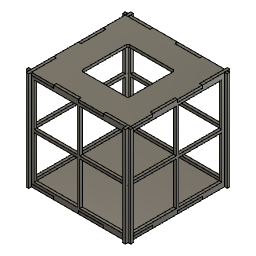
Big Switch Lamp (Autodesk Fusion 360 design; units mm, degrees)
Autodesk Fusion 360 part; units mm, degrees
note: some values were not read from the file. Chosen so that the rebuilt part matches the saved one: which bodies a step acts on.
sketch "Sketch1" plane through (0, 0, 0) normal (1, 0, 0) x (0, 0, -1) in component "Sides"
  line L0 (0, 0) -> (111.6, 0) construction
  line L1 (111.6, 0) -> (111.6, 111.6) construction
  line L2 (111.6, 111.6) -> (0, 111.6) construction
  line L3 (0, 111.6) -> (0, 0) construction
  line L4 (3.175, 108.425) -> (54.2125, 108.425)
  line L5 (54.2125, 108.425) -> (54.2125, 57.3875)
  line L6 (54.2125, 57.3875) -> (3.175, 57.3875)
  line L7 (3.175, 57.3875) -> (3.175, 108.425)
  line L8 (57.3875, 108.425) -> (108.425, 108.425)
  line L9 (108.425, 108.425) -> (108.425, 57.3875)
  line L10 (108.425, 57.3875) -> (57.3875, 57.3875)
  line L11 (57.3875, 57.3875) -> (57.3875, 108.425)
  line L12 (3.175, 54.2125) -> (54.2125, 54.2125)
  line L13 (54.2125, 54.2125) -> (54.2125, 3.175)
  line L14 (54.2125, 3.175) -> (3.175, 3.175)
  line L15 (3.175, 3.175) -> (3.175, 54.2125)
  line L16 (57.3875, 54.2125) -> (108.425, 54.2125)
  line L17 (108.425, 54.2125) -> (108.425, 3.175)
  line L18 (108.425, 3.175) -> (57.3875, 3.175)
  line L19 (57.3875, 3.175) -> (57.3875, 54.2125)
  line L20 (0, 93) -> (3.175, 93) construction
  line L21 (15, 108.425) -> (15, 111.6) construction
  line L22 (15, 57.3875) -> (15, 54.2125) construction
  line L23 (15, 3.175) -> (15, 0) construction
  line L24 (54.2125, 93) -> (57.3875, 93) construction
  line L25 (108.425, 92.9494) -> (111.6, 92.9494) construction
  line L26 (-6.35, 114.775) -> (117.95, 114.775)
  line L27 (117.95, 114.775) -> (117.95, -3.175)
  line L28 (117.95, -3.175) -> (-6.35, -3.175)
  line L29 (-6.35, -3.175) -> (-6.35, 114.775)
  line L30 (108.425, 105.4235) -> (117.95, 105.4235) construction
  line L31 (8.936, 114.775) -> (8.936, 108.425) construction
  dimension "d23" = 111.6
  dimension "d24" = 111.6
  dimension "d25" = 3.175
  dimension "d26" = 3.175
  dimension "d27" = 3.175
  dimension "d28" = 3.175
  dimension "d29" = 3.175
  dimension "d30" = 3.175
  dimension "d31" = 124.3
  dimension "d32" = 9.525
  dimension "d33" = 117.95
  dimension "d34" = 6.35
  constraint horizontal L0
  constraint vertical L1
  constraint horizontal L2
  constraint vertical L3
  constraint coincident L0.start L3.end
  constraint horizontal L4
  constraint vertical L5
  constraint horizontal L6
  constraint vertical L7
  constraint horizontal L8
  constraint vertical L9
  constraint horizontal L10
  constraint vertical L11
  constraint horizontal L12
  constraint vertical L13
  constraint horizontal L14
  constraint vertical L15
  constraint horizontal L16
  constraint vertical L17
  constraint horizontal L18
  constraint vertical L19
  constraint equal L4 L8
  constraint equal L10 L16
  constraint equal L14 L18
  constraint equal L7 L11
  constraint equal L9 L17
  constraint equal L13 L19
  constraint collinear L7 L15
  constraint collinear L11 L19
  constraint collinear L4 L8
  constraint collinear L12 L16
  constraint coincident L3 L20.start
  constraint coincident L7 L20.end
  constraint perpendicular L7 L20
  constraint coincident L4 L21.start
  constraint coincident L2 L21.end
  constraint perpendicular L2 L21
  constraint coincident L6 L22.start
  constraint coincident L12 L22.end
  constraint perpendicular L12 L22
  constraint coincident L14 L23.start
  constraint coincident L0 L23.end
  constraint perpendicular L0 L23
  constraint coincident L5 L24.start
  constraint coincident L11 L24.end
  constraint perpendicular L11 L24
  constraint coincident L9 L25.start
  constraint coincident L1 L25.end
  constraint perpendicular L1 L25
  constraint horizontal L26
  constraint vertical L27
  constraint horizontal L28
  constraint vertical L29
  constraint coincident L9 L30.start
  constraint coincident L27 L30.end
  constraint perpendicular L27 L30
  constraint coincident L26 L31.start
  constraint coincident L4 L31.end
  constraint perpendicular L4 L31
  measures "d23" distance of L0.start L2.end
  measures "d24" distance of L0.start L0.end
  measures "d25" distance of L20.start L20.end
  measures "d26" distance of L24.start L24.end
  measures "d27" distance of L25.start L25.end
  measures "d28" distance of L21.start L21.end
  measures "d29" distance of L22.start L22.end
  measures "d30" distance of L23.start L23.end
  measures "d31" distance of L27.end L28.end
  measures "d32" distance of L30.start L30.end
  measures "d33" distance of L26.start L28.end
  measures "d34" distance of L31.start L31.end
extrude "Extrude1" add sketch "Sketch1" along normal blind 3.175 makes body 1 in component "Sides"
pattern_circular "C-Pattern1" count 4 over 360 about axis through (0, -3.175, 6.35) along (0, 1, 0) of bodies 1 makes body 2 at (-121.125, 56.3292, 6.35) makes body 3 at (0, 56.3292, 127.475) makes body 4 at (121.125, 56.3292, 6.35) in component "Sides"
move_body "Move1" bodies 4 to x (1, 0, 0) y (0, 1, 0) z (0, 0, 1) at (-117.95, 0, -58.975) in component "Sides"
move_body "Move2" bodies 4 to x (1, 0, 0) y (0, 1, 0) z (0, 0, 1) at (0, 0, -62.15) in component "Sides"
move_body "Move3" bodies 2 to x (1, 0, 0) y (0, 1, 0) z (0, 0, 1) at (6.35, 0, -3.175) in component "Sides"
move_body "Move4" bodies 3 to x (1, 0, 0) y (0, 1, 0) z (0, 0, 1) at (-111.6, 0, -124.3) in component "Sides"
sketch "Sketch5" plane through (0, 0, 0) normal (0, 1, 0) x (1, 0, 0) in component "Bottom"
  line L0 (6.35, 114.775) -> (-117.95, 114.775)
  line L1 (-117.95, 114.775) -> (-117.95, 111.6)
  line L2 (-117.95, 111.6) -> (6.35, 111.6) construction
  line L3 (6.35, 111.6) -> (6.35, 114.775)
  line L4 (0, 117.95) -> (0, -6.35) construction
  line L5 (0, -6.35) -> (3.175, -6.35)
  line L6 (3.175, -6.35) -> (3.175, 117.95)
  line L7 (3.175, 117.95) -> (0, 117.95)
  line L8 (-117.95, -3.175) -> (6.35, -3.175)
  line L9 (6.35, -3.175) -> (6.35, 0)
  line L10 (6.35, 0) -> (-117.95, 0) construction
  line L11 (-117.95, 0) -> (-117.95, -3.175)
  line L12 (-111.6, -6.35) -> (-111.6, 117.95) construction
  line L13 (-111.6, 117.95) -> (-114.775, 117.95)
  line L14 (-114.775, 117.95) -> (-114.775, -6.35)
  line L15 (-114.775, -6.35) -> (-111.6, -6.35)
  line L16 (-114.775, 114.775) -> (3.175, 114.775)
  line L17 (3.175, 114.775) -> (3.175, -3.175)
  line L18 (3.175, -3.175) -> (-114.775, -3.175)
  line L19 (-114.775, -3.175) -> (-114.775, 114.775)
  line L20 (-114.775, 114.775) -> (3.175, -3.175) construction
  circle A0 centre (-55.8, 55.8) radius 32.75
  circle A1 centre (-55.8, 55.8) radius 26.1
  line L21 (-68.5, 74.85) -> (-43.1, 74.85)
  line L22 (-43.1, 74.85) -> (-43.1, 36.75)
  line L23 (-43.1, 36.75) -> (-68.5, 36.75)
  line L24 (-68.5, 36.75) -> (-68.5, 74.85)
  line L25 (-68.5, 36.75) -> (-43.1, 74.85) construction
  dimension "d51" = 65.5
  dimension "d52" = 52.2
  dimension "d53" = 25.4
  dimension "d54" = 38.1
  constraint horizontal L16
  constraint vertical L17
  constraint horizontal L18
  constraint vertical L19
  constraint coincident L8 L17.end
  constraint coincident L6 L17.end
  constraint coincident L14 L16.start
  constraint coincident L0 L16.start
  constraint midpoint L20 A0.centre
  constraint horizontal L21
  constraint vertical L22
  constraint horizontal L23
  constraint vertical L24
  constraint midpoint L20 L25
  measures "d51" diameter of A0
  measures "d52" diameter of A1
  measures "d53" distance of L21.start L21.end
  measures "d54" distance of L21.start L23.end
extrude "Extrude4" add sketch "Sketch5" along normal blind 3.175 separate body contours A0 | L21 L22 L23 L24 makes body 5 at (-51.5667, 0, -49.45) makes body 6 at (-25.4858, 0, -52.8763) in component "Bottom"
extrude "Extrude2" add sketch "Sketch5" against normal blind 3.175 separate body contours L0 L6 L8 L14 L16 L17 L18 L19 | A0 | A1 | L21 L22 L23 L24 makes body 7 in component "Bottom"
sketch "Sketch2" plane through (0, 0, 0) normal (0, 1, 0) x (1, 0, 0) in component "Bottom"
  line L0 (6.35, 114.775) -> (-117.95, 114.775)
  line L1 (-117.95, 114.775) -> (-117.95, 111.6)
  line L2 (-117.95, 111.6) -> (6.35, 111.6)
  line L3 (6.35, 111.6) -> (6.35, 114.775)
  line L4 (-111.6, -6.35) -> (-111.6, 117.95)
  line L5 (-111.6, 117.95) -> (-114.775, 117.95)
  line L6 (-114.775, 117.95) -> (-114.775, -6.35)
  line L7 (-114.775, -6.35) -> (-111.6, -6.35)
  line L8 (-117.95, -3.175) -> (6.35, -3.175)
  line L9 (6.35, -3.175) -> (6.35, 0)
  line L10 (6.35, 0) -> (-117.95, 0)
  line L11 (-117.95, 0) -> (-117.95, -3.175)
  line L12 (0, 117.95) -> (0, -6.35)
  line L13 (0, -6.35) -> (3.175, -6.35)
  line L14 (3.175, -6.35) -> (3.175, 117.95)
  line L15 (3.175, 117.95) -> (0, 117.95)
extrude "Extrude3" add sketch "Sketch2" along normal blind 3.175 separate body contours L2 L4 L10 L12 makes body 8 in component "Bottom"
sketch "Sketch2 (2)" plane through (0, 0, 0) normal (0, 1, 0) x (1, 0, 0) in component "Top"
  line L0 (-117.95, -3.175) -> (6.35, -3.175) construction
  line L1 (6.35, -3.175) -> (6.35, 0) construction
  line L2 (6.35, 0) -> (-117.95, 0) construction
  line L3 (-117.95, 0) -> (-117.95, -3.175) construction
  line L4 (0, 117.95) -> (0, -6.35) construction
  line L5 (0, -6.35) -> (3.175, -6.35) construction
  line L6 (3.175, -6.35) -> (3.175, 117.95) construction
  line L7 (3.175, 117.95) -> (0, 117.95) construction
  line L8 (6.35, 114.775) -> (-117.95, 114.775) construction
  line L9 (-117.95, 114.775) -> (-117.95, 111.6) construction
  line L10 (-117.95, 111.6) -> (6.35, 111.6) construction
  line L11 (6.35, 111.6) -> (6.35, 114.775) construction
  line L12 (-111.6, -6.35) -> (-111.6, 117.95) construction
  line L13 (-111.6, 117.95) -> (-114.775, 117.95) construction
  line L14 (-114.775, 117.95) -> (-114.775, -6.35) construction
  line L15 (-114.775, -6.35) -> (-111.6, -6.35) construction
  line L16 (-114.775, 114.775) -> (3.175, 114.775)
  line L17 (3.175, 114.775) -> (3.175, -3.175)
  line L18 (3.175, -3.175) -> (-114.775, -3.175)
  line L19 (-114.775, -3.175) -> (-114.775, 114.775)
  line L20 (3.175, 114.775) -> (-114.775, -3.175) construction
  line L21 (-27.9, 27.9) -> (-83.7, 27.9)
  line L22 (-83.7, 27.9) -> (-83.7, 83.7)
  line L23 (-83.7, 83.7) -> (-27.9, 83.7)
  line L24 (-27.9, 83.7) -> (-27.9, 27.9)
  line L25 (-27.9, 27.9) -> (-83.7, 83.7) construction
  line L26 (-83.7, 27.9) -> (-27.9, 83.7) construction
  line L27 (-114.775, 114.775) -> (-85.2875, 114.775)
  line L28 (-85.2875, 114.775) -> (-85.2875, 111.6)
  line L29 (-85.2875, 111.6) -> (-114.775, 111.6)
  line L30 (-114.775, 111.6) -> (-114.775, 114.775)
  line L31 (-55.8, 114.775) -> (-26.3125, 114.775)
  line L32 (-26.3125, 114.775) -> (-26.3125, 111.6)
  line L33 (-26.3125, 111.6) -> (-55.8, 111.6)
  line L34 (-55.8, 111.6) -> (-55.8, 114.775)
  line L35 (-85.2875, 113.1875) -> (-55.8, 113.1875) construction
  line L36 (-26.3125, 113.1875) -> (3.175, 113.1875) construction
  line L37 (-114.775, 26.3125) -> (-111.6, 26.3125)
  line L38 (-111.6, 55.8) -> (-114.775, 55.8)
  line L39 (-113.1875, 26.3125) -> (-113.1875, 55.8) construction
  line L40 (-111.6, 26.3125) -> (-111.6, -3.175)
  line L41 (-114.775, -3.175) -> (-114.775, 26.3125)
  line L42 (-111.6, -3.175) -> (-114.775, -3.175)
  line L43 (-114.775, 85.2875) -> (-111.6, 85.2875)
  line L44 (-111.6, 85.2875) -> (-111.6, 55.8)
  line L45 (-114.775, 55.8) -> (-114.775, 85.2875)
  line L46 (-26.3125, -3.175) -> (-26.3125, 0)
  line L47 (-55.8, 0) -> (-55.8, -3.175)
  line L48 (-26.3125, -1.5875) -> (-55.8, -1.5875) construction
  line L49 (-26.3125, 0) -> (3.175, 0)
  line L50 (3.175, -3.175) -> (-26.3125, -3.175)
  line L51 (3.175, 0) -> (3.175, -3.175)
  line L52 (-85.2875, -3.175) -> (-85.2875, 0)
  line L53 (-85.2875, 0) -> (-55.8, 0)
  line L54 (-55.8, -3.175) -> (-85.2875, -3.175)
  line L55 (3.175, 85.2875) -> (0, 85.2875)
  line L56 (0, 55.8) -> (3.175, 55.8)
  line L57 (1.5875, 85.2875) -> (1.5875, 55.8) construction
  line L58 (0, 85.2875) -> (0, 114.775)
  line L59 (3.175, 114.775) -> (3.175, 85.2875)
  line L60 (0, 114.775) -> (3.175, 114.775)
  line L61 (3.175, 26.3125) -> (0, 26.3125)
  line L62 (0, 26.3125) -> (0, 55.8)
  line L63 (3.175, 55.8) -> (3.175, 26.3125)
  point P0 (-55.8, 55.8)
  point P1 (-113.1875, 85.2875)
  point P2 (-85.2875, -1.5875)
  point P3 (1.5875, 26.3125)
  dimension "d47" = 55.8
  dimension "d48" = 55.8
  dimension "d68" = 360
  constraint horizontal L16
  constraint vertical L17
  constraint horizontal L18
  constraint vertical L19
  constraint coincident L0 L17.end
  constraint coincident L6 L17.end
  constraint coincident L8 L16.start
  constraint coincident L14 L16.start
  constraint perpendicular L21 L22
  constraint parallel L21 L23
  constraint parallel L22 L24
  constraint horizontal L21
  constraint coincident L25 P0
  constraint coincident L26 P0
  constraint midpoint L20 P0
  constraint horizontal L27
  constraint vertical L28
  constraint horizontal L29
  constraint vertical L30
  constraint coincident L10 L28.end
  constraint horizontal L31
  constraint vertical L32
  constraint horizontal L33
  constraint vertical L34
  constraint coincident L10 L32.end
  constraint coincident L8 L31.start
  constraint midpoint L28 L35.start
  constraint midpoint L34 L35.end
  constraint midpoint L32 L36.start
  constraint coincident L6 L36.end
  constraint horizontal L36
  constraint equal L27 L35
  constraint equal L33 L35
  constraint equal L33 L36
  measures "d47" distance of L22.end L23.end
  measures "d48" distance of L21.end L22.end
extrude "Extrude2'" add sketch "Sketch2 (2)" along normal blind 3.175 separate body makes body 9 in component "Top"
move_body "Move2'" bodies 9 to x (1, 0, 0) y (0, 1, 0) z (0, 0, 1) at (0, 111.6, 0) in component "Top"
combine "Combine1" operation cut target body 8 tool bodies 5 6 makes body 10 at (-56.6158, 0, -7.7139) in component "Bottom"
fillet "Fillet1" radius 2 4 edges at (-83.7, 113.1875, -83.7) (-27.9, 113.1875, -83.7) (-27.9, 113.1875, -27.9) (-83.7, 113.1875, -27.9) on bodies 9 in component "Top"
sketch "Sketch7" plane through (0, 0, 3.175) normal (0, 0, 1) x (1, 0, 0) in component "Sides"
  line L0 (-3.175, 3.175) -> (-54.2125, 3.175)
  line L1 (-54.2125, 3.175) -> (-54.2125, 54.2125)
  line L2 (-54.2125, 54.2125) -> (-3.175, 54.2125)
  line L3 (-3.175, 54.2125) -> (-3.175, 3.175)
  line L4 (-57.3875, 3.175) -> (-108.425, 3.175)
  line L5 (-108.425, 3.175) -> (-108.425, 54.2125)
  line L6 (-108.425, 54.2125) -> (-57.3875, 54.2125)
  line L7 (-57.3875, 54.2125) -> (-57.3875, 3.175)
  line L8 (-57.3875, 57.3875) -> (-108.425, 57.3875)
  line L9 (-108.425, 57.3875) -> (-108.425, 108.425)
  line L10 (-108.425, 108.425) -> (-57.3875, 108.425)
  line L11 (-57.3875, 108.425) -> (-57.3875, 57.3875)
  line L12 (-3.175, 57.3875) -> (-54.2125, 57.3875)
  line L13 (-54.2125, 57.3875) -> (-54.2125, 108.425)
  line L14 (-54.2125, 108.425) -> (-3.175, 108.425)
  line L15 (-3.175, 108.425) -> (-3.175, 57.3875)
  line L16 (-117.95, -3.175) -> (6.35, -3.175)
  line L17 (6.35, -3.175) -> (6.35, 114.775)
  line L18 (6.35, 114.775) -> (-117.95, 114.775)
  line L19 (-117.95, 114.775) -> (-117.95, -3.175)
  line L20 (0, 114.775) -> (0, -3.175) construction
  line L21 (0, -3.175) -> (3.175, -3.175) construction
  line L22 (3.175, -3.175) -> (3.175, 114.775) construction
  line L23 (3.175, 114.775) -> (0, 114.775) construction
  line L24 (-111.6, -3.175) -> (-111.6, 114.775) construction
  line L25 (-111.6, 114.775) -> (-114.775, 114.775) construction
  line L26 (-114.775, 114.775) -> (-114.775, -3.175) construction
  line L27 (-114.775, -3.175) -> (-111.6, -3.175) construction
  line L28 (0, 114.775) -> (3.175, 114.775)
  line L29 (3.175, 114.775) -> (3.175, 55.8)
  line L30 (3.175, 55.8) -> (0, 55.8)
  line L31 (0, 55.8) -> (0, 114.775)
  line L32 (-114.775, 55.8) -> (-111.6, 55.8)
  line L33 (-111.6, 55.8) -> (-111.6, 114.775)
  line L34 (-111.6, 114.775) -> (-114.775, 114.775)
  line L35 (-114.775, 114.775) -> (-114.775, 55.8)
  line L36 (3.175, 0) -> (-114.775, 0) construction
  line L37 (-114.775, 0) -> (-114.775, -3.175) construction
  line L38 (-114.775, -3.175) -> (3.175, -3.175) construction
  line L39 (3.175, -3.175) -> (3.175, 0) construction
  constraint horizontal L28
  constraint vertical L29
  constraint horizontal L30
  constraint vertical L31
  constraint midpoint L22 L29.end
  constraint coincident L20.start L23.end
  constraint horizontal L32
  constraint vertical L33
  constraint horizontal L34
  constraint vertical L35
  constraint coincident L24.end L25.start
  constraint midpoint L26 L32.start
extrude "Extrude2''" cut sketch "Sketch7" against normal blind 3.175 contours L18 L32 L33 L34 L35 | L18 L28 L29 L30 L31 bodies 2 in component "Sides"
combine "Combine1'" operation cut target body 3 tool bodies 2 keep tools in component "Sides"
combine "Combine2" operation cut target body 1 tool bodies 2 keep tools in component "Sides"
sketch "Sketch8" plane through (0, 0, -111.6) normal (0, 0, 1) x (1, 0, 0) in component "Sides"
  line L0 (-57.3875, 3.175) -> (-108.425, 3.175)
  line L1 (-108.425, 3.175) -> (-108.425, 54.2125)
  line L2 (-108.425, 54.2125) -> (-57.3875, 54.2125)
  line L3 (-57.3875, 54.2125) -> (-57.3875, 3.175)
  line L4 (-3.175, 3.175) -> (-54.2125, 3.175)
  line L5 (-54.2125, 3.175) -> (-54.2125, 54.2125)
  line L6 (-54.2125, 54.2125) -> (-3.175, 54.2125)
  line L7 (-3.175, 54.2125) -> (-3.175, 3.175)
  line L8 (-3.175, 57.3875) -> (-54.2125, 57.3875)
  line L9 (-54.2125, 57.3875) -> (-54.2125, 108.425)
  line L10 (-54.2125, 108.425) -> (-3.175, 108.425)
  line L11 (-3.175, 108.425) -> (-3.175, 57.3875)
  line L12 (-57.3875, 57.3875) -> (-108.425, 57.3875)
  line L13 (-108.425, 57.3875) -> (-108.425, 108.425)
  line L14 (-108.425, 108.425) -> (-57.3875, 108.425)
  line L15 (-57.3875, 108.425) -> (-57.3875, 57.3875)
  line L16 (-117.95, -3.175) -> (6.35, -3.175)
  line L17 (6.35, -3.175) -> (6.35, 114.775)
  line L18 (6.35, 114.775) -> (-117.95, 114.775)
  line L19 (-117.95, 114.775) -> (-117.95, -3.175)
  line L20 (0, 55.8) -> (0, 114.775) construction
  line L21 (0, 114.775) -> (-111.6, 114.775) construction
  line L22 (-111.6, 114.775) -> (-111.6, 55.8) construction
  line L23 (-111.6, 55.8) -> (-114.775, 55.8) construction
  line L24 (-114.775, 55.8) -> (-114.775, 114.775) construction
  line L25 (-114.775, 114.775) -> (-117.95, 114.775) construction
  line L26 (-117.95, 114.775) -> (-117.95, -3.175) construction
  line L27 (-117.95, -3.175) -> (6.35, -3.175) construction
  line L28 (6.35, -3.175) -> (6.35, 114.775) construction
  line L29 (6.35, 114.775) -> (3.175, 114.775) construction
  line L30 (3.175, 114.775) -> (3.175, 55.8) construction
  line L31 (3.175, 55.8) -> (0, 55.8) construction
  line L32 (-3.175, 3.175) -> (-54.2125, 3.175) construction
  line L33 (-54.2125, 3.175) -> (-54.2125, 54.2125) construction
  line L34 (-54.2125, 54.2125) -> (-3.175, 54.2125) construction
  line L35 (-3.175, 54.2125) -> (-3.175, 3.175) construction
  line L36 (-57.3875, 3.175) -> (-108.425, 3.175) construction
  line L37 (-108.425, 3.175) -> (-108.425, 54.2125) construction
  line L38 (-108.425, 54.2125) -> (-57.3875, 54.2125) construction
  line L39 (-57.3875, 54.2125) -> (-57.3875, 3.175) construction
  line L40 (-57.3875, 57.3875) -> (-108.425, 57.3875) construction
  line L41 (-108.425, 57.3875) -> (-108.425, 108.425) construction
  line L42 (-108.425, 108.425) -> (-57.3875, 108.425) construction
  line L43 (-57.3875, 108.425) -> (-57.3875, 57.3875) construction
  line L44 (-3.175, 57.3875) -> (-54.2125, 57.3875) construction
  line L45 (-54.2125, 57.3875) -> (-54.2125, 108.425) construction
  line L46 (-54.2125, 108.425) -> (-3.175, 108.425) construction
  line L47 (-3.175, 108.425) -> (-3.175, 57.3875) construction
  line L48 (-114.775, 114.775) -> (-111.6, 114.775)
  line L49 (-111.6, 114.775) -> (-111.6, 55.8)
  line L50 (-111.6, 55.8) -> (-114.775, 55.8)
  line L51 (-114.775, 55.8) -> (-114.775, 114.775)
  line L52 (0, 114.775) -> (3.175, 114.775)
  line L53 (3.175, 114.775) -> (3.175, 55.8)
  line L54 (3.175, 55.8) -> (0, 55.8)
  line L55 (0, 55.8) -> (0, 114.775)
  constraint horizontal L48
  constraint vertical L49
  constraint horizontal L50
  constraint vertical L51
  constraint coincident L22.end L23.start
  constraint coincident L24.end L25.start
  constraint horizontal L52
  constraint vertical L53
  constraint horizontal L54
  constraint vertical L55
  constraint coincident L30.end L31.start
  constraint coincident L20.end L21.start
extrude "Extrude3'" cut sketch "Sketch8" against normal blind 3.175 contours L18 L48 L49 L50 L51 | L18 L52 L53 L54 L55 bodies 4 in component "Sides"
combine "Combine3" operation cut target body 3 tool bodies 4 keep tools in component "Sides"
combine "Combine4" operation cut target body 1 tool bodies 4 keep tools in component "Sides"
sketch "Sketch4" plane through (0, 0, 0) normal (0, 1, 0) x (-1, 0, 0) in component "Bottom"
  line L0 (114.775, 3.175) -> (-3.175, 3.175)
  line L1 (-3.175, 3.175) -> (-3.175, -114.775)
  line L2 (-3.175, -114.775) -> (114.775, -114.775)
  line L3 (114.775, -114.775) -> (114.775, 3.175)
  line L4 (111.6, 6.35) -> (111.6, -117.95) construction
  line L5 (111.6, -117.95) -> (114.775, -117.95) construction
  line L6 (114.775, -117.95) -> (114.775, 6.35) construction
  line L7 (114.775, 6.35) -> (111.6, 6.35) construction
  line L8 (0, -117.95) -> (0, 6.35) construction
  line L9 (0, 6.35) -> (-3.175, 6.35) construction
  line L10 (-3.175, 6.35) -> (-3.175, -117.95) construction
  line L11 (-3.175, -117.95) -> (0, -117.95) construction
  line L12 (0, 3.175) -> (0, 0) construction
  line L13 (0, 0) -> (111.6, 0) construction
  line L14 (111.6, 0) -> (111.6, 3.175) construction
  line L15 (111.6, 3.175) -> (0, 3.175) construction
  line L16 (0, -111.6) -> (0, -114.775) construction
  line L17 (0, -114.775) -> (111.6, -114.775) construction
  line L18 (111.6, -114.775) -> (111.6, -111.6) construction
  line L19 (111.6, -111.6) -> (0, -111.6) construction
  line L20 (114.775, -114.775) -> (85.2875, -114.775)
  line L21 (85.2875, -114.775) -> (85.2875, -111.6)
  line L22 (85.2875, -111.6) -> (114.775, -111.6)
  line L23 (114.775, -111.6) -> (114.775, -114.775)
  line L24 (55.8, -114.775) -> (26.3125, -114.775)
  line L25 (26.3125, -114.775) -> (26.3125, -111.6)
  line L26 (26.3125, -111.6) -> (55.8, -111.6)
  line L27 (55.8, -111.6) -> (55.8, -114.775)
  line L28 (85.2875, -113.1875) -> (55.8, -113.1875) construction
  line L29 (26.3125, -113.1875) -> (-3.175, -113.1875) construction
  line L30 (114.775, -114.775) -> (-3.175, 3.175) construction
  line L31 (114.775, 3.175) -> (-3.175, -114.775) construction
  line L32 (114.775, -55.8) -> (114.775, -85.2875)
  line L33 (114.775, -85.2875) -> (111.6, -85.2875)
  line L34 (111.6, -26.3125) -> (111.6, 3.175)
  line L35 (113.1875, -26.3125) -> (113.1875, -55.8) construction
  line L36 (111.6, -85.2875) -> (111.6, -55.8)
  line L37 (111.6, 3.175) -> (114.775, 3.175)
  line L38 (111.6, -55.8) -> (114.775, -55.8)
  line L39 (114.775, 3.175) -> (114.775, -26.3125)
  line L40 (114.775, -26.3125) -> (111.6, -26.3125)
  line L41 (114.775, 0) -> (111.6, 0) construction
  line L42 (55.8, 3.175) -> (85.2875, 3.175)
  line L43 (85.2875, 3.175) -> (85.2875, 0)
  line L44 (26.3125, 0) -> (-3.175, 0)
  line L45 (26.3125, 1.5875) -> (55.8, 1.5875) construction
  line L46 (85.2875, 0) -> (55.8, 0)
  line L47 (-3.175, 0) -> (-3.175, 3.175)
  line L48 (55.8, 0) -> (55.8, 3.175)
  line L49 (-3.175, 3.175) -> (26.3125, 3.175)
  line L50 (26.3125, 3.175) -> (26.3125, 0)
  line L51 (0, 3.175) -> (0, 0) construction
  line L52 (-3.175, -55.8) -> (-3.175, -26.3125)
  line L53 (-3.175, -26.3125) -> (0, -26.3125)
  line L54 (0, -85.2875) -> (0, -114.775)
  line L55 (-1.5875, -85.2875) -> (-1.5875, -55.8) construction
  line L56 (0, -26.3125) -> (0, -55.8)
  line L57 (0, -114.775) -> (-3.175, -114.775)
  line L58 (0, -55.8) -> (-3.175, -55.8)
  line L59 (-3.175, -114.775) -> (-3.175, -85.2875)
  line L60 (-3.175, -85.2875) -> (0, -85.2875)
  line L61 (-3.175, -111.6) -> (0, -111.6) construction
  point P0 (55.8, -55.8)
  point P1 (113.1875, -85.2875)
  point P2 (114.775, 3.175)
  point P3 (85.2875, 1.5875)
  point P4 (-3.175, 3.175)
  point P5 (-1.5875, -26.3125)
  point P6 (-3.175, -114.775)
  dimension "d64" = 360
  constraint horizontal L20
  constraint vertical L21
  constraint horizontal L22
  constraint vertical L23
  constraint coincident L19 L21.end
  constraint coincident L2.end L3.start
  constraint horizontal L24
  constraint vertical L25
  constraint horizontal L26
  constraint vertical L27
  constraint coincident L19 L25.end
  constraint coincident L17 L24.start
  constraint equal L20 L24
  constraint midpoint L21 L28.start
  constraint midpoint L27 L28.end
  constraint equal L20 L28
  constraint midpoint L25 L29.start
  constraint coincident L1 L29.end
  constraint horizontal L29
  constraint equal L24 L29
  constraint coincident P4 L0.end
  constraint coincident P2 L0.start
  constraint coincident P6 L1.end
  constraint midpoint L31 P0
extrude "Extrude5" cut sketch "Sketch4" against normal blind 3.175 contours L0 L3 L34 L37 L39 L40 | L0 L42 L43 L46 L48 | L3 L32 L33 L36 L38 | L0 L1 L44 L47 L49 L50 | L2 L3 L20 L21 L22 L23 | L1 L52 L53 L56 L58 | L2 L24 L25 L26 L27 | L1 L2 L54 L57 L59 L60 bodies 7 in component "Bottom"
combine "Combine5" operation cut target body 2 tool bodies 7 keep tools in component "Sides"
combine "Combine6" operation cut target body 1 tool bodies 7 keep tools in component "Sides"
combine "Combine7" operation cut target body 3 tool bodies 7 keep tools in component "Sides"
combine "Combine8" operation cut target body 4 tool bodies 7 keep tools in component "Sides"
sketch "Sketch3" plane through (0, 114.775, 0) normal (0, 1, 0) x (-1, 0, 0) in component "Top"
  line L0 (81.7, -83.7) -> (29.9, -83.7)
  arc A0 (27.9, -81.7) -> (29.9, -83.7) centre (29.9, -81.7) ccw
  line L1 (27.9, -81.7) -> (27.9, -29.9)
  arc A1 (29.9, -27.9) -> (27.9, -29.9) centre (29.9, -29.9) ccw
  line L2 (29.9, -27.9) -> (81.7, -27.9)
  arc A2 (83.7, -29.9) -> (81.7, -27.9) centre (81.7, -29.9) ccw
  line L3 (83.7, -29.9) -> (83.7, -81.7)
  arc A3 (81.7, -83.7) -> (83.7, -81.7) centre (81.7, -81.7) ccw
  line L4 (114.775, 3.175) -> (-3.175, 3.175)
  line L5 (-3.175, 3.175) -> (-3.175, -114.775)
  line L6 (-3.175, -114.775) -> (114.775, -114.775)
  line L7 (114.775, -114.775) -> (114.775, 3.175)
  line L8 (85.2875, 0) -> (85.2875, 3.175)
  line L9 (55.8, 3.175) -> (55.8, 0)
  line L10 (55.8, 0) -> (85.2875, 0)
  line L11 (26.3125, -111.6) -> (26.3125, -114.775)
  line L12 (55.8, -114.775) -> (55.8, -111.6)
  line L13 (55.8, -111.6) -> (26.3125, -111.6)
  line L14 (0, -114.775) -> (0, -85.2875)
  line L15 (0, -85.2875) -> (-3.175, -85.2875)
  line L16 (111.6, 3.175) -> (111.6, -26.3125)
  line L17 (111.6, -26.3125) -> (114.775, -26.3125)
  line L18 (-3.175, 0) -> (26.3125, 0)
  line L19 (26.3125, 0) -> (26.3125, 3.175)
  line L20 (85.2875, -111.6) -> (85.2875, -114.775)
  line L21 (114.775, -111.6) -> (85.2875, -111.6)
  line L22 (0, -26.3125) -> (-3.175, -26.3125)
  line L23 (-3.175, -55.8) -> (0, -55.8)
  line L24 (0, -55.8) -> (0, -26.3125)
  line L25 (111.6, -85.2875) -> (114.775, -85.2875)
  line L26 (114.775, -55.8) -> (111.6, -55.8)
  line L27 (111.6, -55.8) -> (111.6, -85.2875)
  line L28 (85.2875, 3.175) -> (111.6, 3.175)
  line L29 (26.3125, -114.775) -> (0, -114.775)
  line L30 (-3.175, -26.3125) -> (-3.175, 0)
  line L31 (114.775, -26.3125) -> (114.775, -55.8)
  line L32 (114.775, -85.2875) -> (114.775, -111.6)
  line L33 (85.2875, -114.775) -> (55.8, -114.775)
  line L34 (-3.175, -85.2875) -> (-3.175, -55.8)
  line L35 (26.3125, 3.175) -> (55.8, 3.175)
extrude "Extrude3''" cut sketch "Sketch3" against normal blind 3.175 contours L4 L7 L16 L17 | L4 L8 L9 L10 | L7 L25 L26 L27 | L4 L5 L18 L19 | L6 L7 L20 L21 | L5 L22 L23 L24 | L6 L11 L12 L13 | L5 L6 L14 L15 bodies 9 in component "Top"
combine "Combine9" operation cut target body 1 tool bodies 9 keep tools in component "Sides"
combine "Combine10" operation cut target body 2 tool bodies 9 keep tools in component "Sides"
combine "Combine11" operation cut target body 3 tool bodies 9 keep tools in component "Sides"
combine "Combine12" operation cut target body 4 tool bodies 9 keep tools in component "Sides"
component "Bottom" placed x (1, 0, 0) y (0, 1, 0) z (0, 0, 1) at (0, 0, 0)
component "Sides" placed x (1, 0, 0) y (0, 1, 0) z (0, 0, 1) at (0, 0, 0)
component "Top" placed x (1, 0, 0) y (0, 1, 0) z (0, 0, 1) at (0, 0, 0)
hidden bodies 8 10
equation "base = 55.8 mm"
equation "t = ( 1 / 8 ) * 1 in"
equation "d23 = 2 * base"
equation "d24 = 2 * base"
equation "d25 = t"
equation "d26 = t"
equation "d27 = t"
equation "d28 = t"
equation "d29 = t"
equation "d30 = t"
equation "d31 = 2 * base + 4 * t"
equation "d32 = 3 * t"
equation "d33 = 2 * base + 2 * t"
equation "d34 = 2 * t"
equation "d35 = t"
equation "d39 = -t"
equation "d41 = t"
equation "d47 = base"
equation "d48 = base"
equation "d49 = t"
equation "d55 = t"
equation "d58 = -t"
equation "d60 = -t"
equation "d65 = -t"
equation "d69 = -t"
named bodies: "Right", "Front", "Left", "Back", "Bottom", "Inside Mount", "Top", "Outside Mount"
